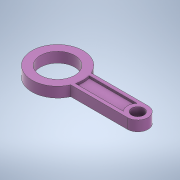
# Autodesk Inventor part: 偏心轮外连接件
Saved by Autodesk Inventor 2022 (Build 260153000, 153)
## iProperties
Created: 2022-05-21
Part Number: 偏心轮外连接件
Material: 常规
Document SubType Name: Modeling
Designer: zhcne
Density: 1 g/cm^3
Appearance: 默认
Author: zhcne
Autodesk Inventor part; units mm, degrees
ref_plane "XZ Plane" through (0, 0, 0) normal (0, 1, 0) x (-1, 0, 0)
ref_plane "XY Plane" through (0, 0, 0) normal (0, 0, 1) x (1, 0, 0)
sketch "草图1" plane through (0, 0, 0) normal (0, 1, 0) x (-1, 0, 0)
  circle A0 centre (0, 0) radius 10.1
  circle A1 centre (0, 0) radius 15
  dimension "d0" = 20.2
  dimension "d1" = 30
  constraints: 2 centre point, 2 coincident
  measures "d0" diameter of A0
  measures "d1" diameter of A1
extrude "拉伸1" add sketch "草图1" along normal blind 6
ref_plane "工作平面1" through (12, 0, 0) normal (1, 0, 0) x (0, 1, 0)
sketch "草图2" plane through (12, 0, 0) normal (1, 0, 0) x (0, 1, 0)
  line L0 (6, -15) -> (6, 15) construction
  line L1 (6, -6) -> (0, -6)
  line L2 (0, -6) -> (0, 6) construction
  line L3 (0, -15) -> (0, 15) construction
  line L4 (6, 6) -> (6, -6) construction
  line L5 (0, 6) -> (6, 6)
  line L6 (6, 0) -> (0, 0)
  line L7 (6, 6) -> (6, 4)
  line L8 (6, 4) -> (4.75, 4)
  line L9 (4.75, 4) -> (4.75, -4)
  line L10 (4.75, -4) -> (6, -4)
  line L11 (6, -4) -> (6, -6)
  line L12 (0, -6) -> (0, -4)
  line L13 (1.25, -4) -> (0, -4)
  line L14 (1.25, -4) -> (1.25, 4)
  line L15 (1.25, 4) -> (0, 4)
  line L16 (0, 6) -> (0, 4)
  line L17 (3, 6) -> (3, -6)
  dimension "d5" = 12
  dimension "d6" = 2
  dimension "d7" = 3.5
  constraints: 32 end point, 6 point on line, 5 collinear, 5 horizontal, 4 perpendicular, 3 midpoint, 1 vertical, 2 other
  measures "d5" distance between parallel lines of L1 L5
  measures "d6" distance between parallel lines of L1 L10
  measures "d7" distance between parallel lines of L14 L9
extrude "拉伸2" add sketch "草图2" along normal blind 35
sketch "草图3" plane through (0, 0, 0) normal (0, 1, 0) x (-1, 0, 0)
  line L0 (-47, 4) -> (-47, -4) projected
  circle A0 centre (-47, 0) radius 6
  circle A1 centre (-47, 0) radius 3.6
  point P0 (0, 0)
  point P1 (-47, -6)
  dimension "d10" = 7.2
  constraints: 1 centre point, 1 coincident, 1 midpoint, 1 vertical alignment, 2 other
  measures "d10" diameter of A1
extrude "拉伸3" cut sketch "草图3" along normal mid plane 35 contours A1 L0 | L0 A1
extrude "拉伸4" add sketch "草图3" along normal blind 6
